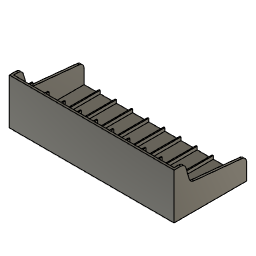
Oblig2Fusion360 (Autodesk Fusion 360 design; units mm, degrees)
Autodesk Fusion 360 part; units mm, degrees
note: some values were not read from the file. Chosen so that the rebuilt part matches the saved one: which face or edge a step refers to. Set by a fixed rule: which sketch regions a step uses.
sketch "Sketch1" plane through (0, 0, 0) normal (0, 0, 1) x (1, 0, 0)
  line L0 (2, 2) -> (172, 2)
  line L1 (172, 2) -> (172, 137)
  line L2 (172, 137) -> (2, 137)
  line L3 (2, 137) -> (2, 2)
  dimension "d1" = 170
  dimension "d2" = 135
  constraint horizontal L0
  constraint vertical L1
  constraint horizontal L2
  constraint vertical L3
  measures "d1" distance of L0.start L0.end
  measures "d2" distance of L0.start L2.end
sketch "Sketch2" plane through (0, 0, 0) normal (0, 0, 1) x (1, 0, 0)
  line L0 (10, 10) -> (158, 10)
  line L1 (158, 10) -> (158, 77.5)
  line L2 (158, 77.5) -> (10, 77.5)
  line L3 (10, 77.5) -> (10, 10)
  dimension "d5" = 148
  dimension "d6" = 67.5
  constraint horizontal L0
  constraint vertical L1
  constraint horizontal L2
  constraint vertical L3
  measures "d5" distance of L0.start L0.end
  measures "d6" distance of L0.start L2.end
extrude "Extrude2" add sketch "Sketch2" along normal blind 42.5
sketch "Sketch3" plane through (158, 0, 0) normal (1, 0, 0) x (0, 1, 0)
  line L0 (10, 0) -> (77.5, 0)
  line L1 (77.5, 0) -> (77.5, 42.5)
  line L2 (77.5, 42.5) -> (10, 42.5)
  line L3 (10, 42.5) -> (10, 0)
  line L4 (10, 42.5) -> (16.2285, 42.5)
  line L5 (28.3819, 24.6655) -> (72.9921, 20.2531)
  line L6 (24.0664, 28.2676) -> (21.0361, 38.8736)
  line L7 (10, 42.5) -> (10, 0)
  line L8 (77.5, 0) -> (77.5, 15.2774)
  line L9 (77.5, 0) -> (10, 0)
  arc A0 (77.5, 15.2774) -> (72.9921, 20.2531) centre (72.5, 15.2774) ccw
  arc A1 (21.0361, 38.8736) -> (16.2285, 42.5) centre (16.2285, 37.5) ccw
  arc A2 (24.0664, 28.2676) -> (28.3819, 24.6655) centre (28.874, 29.6412) ccw
  dimension "d9" = 5
  constraint coincident L2.end L3.start
  constraint perpendicular L3 L4
  constraint coincident L0.start L3.end
  constraint coincident L0.end L1.start
  constraint tangent L5 A0
  constraint tangent L8 A0
  constraint tangent L4 A1
  constraint tangent L6 A1
  constraint equal A0 A1
  constraint tangent L6 A2
  constraint tangent L5 A2
  constraint equal A0 A2
  measures "d9" radius of A0
extrude "Extrude3" cut sketch "Sketch3" against normal blind 150 contours L1 L2 L5 L6 A0 A1 A2
extrude "Extrude4" add 1 faces at (158, 38.6273, 8.2218) along direction (1, 0, 0) blind 4
sketch "Sketch4" plane through (0, 77.5, 0) normal (0, 1, 0) x (-1, 0, 0)
  line L0 (-10, 15.2774) -> (-162, 15.2774)
  line L1 (-162, 15.2774) -> (-162, 0)
  line L2 (-162, 0) -> (-10, 0)
  line L3 (-10, 0) -> (-10, 15.2774)
  line L4 (-162, 15.2774) -> (-160, 15.2774)
  line L5 (-160, 15.2774) -> (-160, 0)
  line L6 (-160, 0) -> (-162, 0)
  line L7 (-162, 0) -> (-162, 15.2774)
  line L8 (-162, 15.2774) -> (-160, 15.2774)
  line L9 (-160, 15.2774) -> (-160, 86.9563)
  line L10 (-160, 86.9563) -> (-162, 86.9563)
  line L11 (-162, 86.9563) -> (-162, 15.2774)
  line L12 (-10, 0) -> (-12, 0)
  line L13 (-12, 0) -> (-12, 80)
  line L14 (-12, 80) -> (-10, 80)
  line L15 (-10, 80) -> (-10, 0)
  line L16 (-160, 0) -> (-12, 0)
  line L17 (-12, 0) -> (-12, 80)
  line L18 (-12, 80) -> (-160, 80)
  line L19 (-160, 80) -> (-160, 0)
  dimension "d14" = 2
  constraint horizontal L4
  constraint vertical L5
  constraint horizontal L6
  constraint vertical L7
  constraint coincident L0.end L1.start
  constraint horizontal L8
  constraint vertical L9
  constraint horizontal L10
  constraint vertical L11
  constraint horizontal L12
  constraint vertical L13
  constraint horizontal L14
  constraint vertical L15
  constraint coincident L2.end L3.start
  constraint horizontal L16
  constraint vertical L17
  constraint horizontal L18
  constraint vertical L19
  measures "d14" distance of L0.end L4.end
extrude "Extrude5" cut sketch "Sketch4" against normal blind 65.5 contours L0 L9 L13 L17 L18 L19
sketch "Sketch5" plane through (0, 77.5, 0) normal (0, 1, 0) x (-1, 0, 0)
  line L0 (-10, 15.2774) -> (-12, 15.2774)
  line L1 (-12, 15.2774) -> (-160, 15.2774)
  line L2 (-160, 15.2774) -> (-162, 15.2774)
  line L3 (-162, 15.2774) -> (-162, 0)
  line L4 (-162, 0) -> (-10, 0)
  line L5 (-10, 0) -> (-10, 15.2774)
  line L6 (-162, 15.2774) -> (-160, 15.2774)
  line L7 (-160, 15.2774) -> (-160, 0)
  line L8 (-160, 0) -> (-162, 0)
  line L9 (-162, 0) -> (-162, 15.2774)
  line L10 (-10, 15.2774) -> (-12, 15.2774)
  line L11 (-12, 15.2774) -> (-12, 0)
  line L12 (-12, 0) -> (-10, 0)
  line L13 (-10, 0) -> (-10, 15.2774)
  line L14 (-160, 15.2774) -> (-12, 15.2774)
  line L15 (-12, 15.2774) -> (-12, 0)
  line L16 (-12, 0) -> (-160, 0)
  line L17 (-160, 0) -> (-160, 15.2774)
  constraint horizontal L6
  constraint vertical L7
  constraint horizontal L8
  constraint vertical L9
  constraint coincident L4 L7.end
  constraint coincident L2.end L3.start
  constraint horizontal L10
  constraint vertical L11
  constraint horizontal L12
  constraint vertical L13
  constraint coincident L4 L11.end
  constraint coincident L0.start L5.end
  constraint horizontal L14
  constraint vertical L15
  constraint horizontal L16
  constraint vertical L17
  constraint coincident L1.end L2.start
extrude "Extrude6" cut sketch "Sketch5" against normal blind 65.5 contours L1 L4 L7 L11 L14 L15 L16 L17
sketch "Sketch6" plane through (0, 0, 0) normal (0, 0, 1) x (1, 0, 0)
  line L0 (12, 12) -> (160, 12)
  line L1 (160, 12) -> (160, 77.5)
  line L2 (160, 77.5) -> (12, 77.5)
  line L3 (12, 77.5) -> (12, 12)
  constraint horizontal L0
  constraint vertical L1
  constraint horizontal L2
  constraint vertical L3
extrude "Extrude7" add sketch "Sketch6" along normal blind 2
extrude "Extrude8" add 1 faces at (61.3333, 55.6667, 2) along direction (0, 0, 1) blind 3
sketch "Sketch7" plane through (0, 0, 5) normal (0, 0, 1) x (-1, 0, 0)
  line L0 (-12, -77.5) -> (-12, -12)
  line L1 (-12, -12) -> (-160, -12)
  line L2 (-160, -12) -> (-160, -77.5)
  line L3 (-160, -77.5) -> (-12, -77.5)
  line L4 (-160, -77.5) -> (-146, -77.5)
  line L5 (-146, -77.5) -> (-146, -12)
  line L6 (-146, -12) -> (-160, -12)
  line L7 (-160, -12) -> (-160, -77.5)
  dimension "d24" = 14
  dimension "d25" = 65.5
  constraint horizontal L4
  constraint vertical L5
  constraint horizontal L6
  constraint vertical L7
  constraint coincident L2.end L3.start
  measures "d24" distance of L2.end L4.end
  measures "d25" distance of L2.end L1.end
extrude "Extrude9" cut sketch "Sketch7" against normal blind 3 contours L1 L2 L3 L4 L5 L6 L7
sketch "Sketch8" plane through (0, 0, 5) normal (0, 0, 1) x (-1, 0, 0)
  line L0 (-146, -12) -> (-146, -77.5)
  line L1 (-146, -77.5) -> (-12, -77.5)
  line L2 (-12, -77.5) -> (-12, -12)
  line L3 (-12, -12) -> (-146, -12)
  line L4 (-146, -77.5) -> (-145, -77.5)
  line L5 (-145, -77.5) -> (-145, -12)
  line L6 (-145, -12) -> (-146, -12)
  line L7 (-146, -12) -> (-146, -77.5)
  line L8 (-145, -77.5) -> (-131, -77.5)
  line L9 (-131, -77.5) -> (-131, -12)
  line L10 (-131, -12) -> (-145, -12)
  line L11 (-145, -12) -> (-145, -77.5)
  line L12 (-131, -77.5) -> (-130, -77.5)
  line L13 (-130, -77.5) -> (-130, -12)
  line L14 (-130, -12) -> (-131, -12)
  line L15 (-131, -12) -> (-131, -77.5)
  dimension "d28" = 1
  dimension "d29" = 65.5
  dimension "d30" = 14
  dimension "d31" = 65.5
  dimension "d32" = 1
  dimension "d33" = 65.5
  constraint horizontal L4
  constraint vertical L5
  constraint horizontal L6
  constraint vertical L7
  constraint coincident L0.end L1.start
  constraint horizontal L8
  constraint vertical L9
  constraint horizontal L10
  constraint vertical L11
  constraint horizontal L12
  constraint vertical L13
  constraint horizontal L14
  constraint vertical L15
  measures "d28" distance of L0.end L4.end
  measures "d29" distance of L0.end L0.start
  measures "d30" distance of L4.end L8.end
  measures "d31" distance of L4.end L5.end
  measures "d32" distance of L8.end L12.end
  measures "d33" distance of L8.end L9.end
extrude "Extrude10" cut sketch "Sketch8" against normal blind 3 contours L1 L3 L5 L8 L9 L10 L11 L15
sketch "Sketch9" plane through (0, 0, 5) normal (0, 0, 1) x (-1, 0, 0)
  line L0 (-131, -12) -> (-131, -77.5)
  line L1 (-131, -77.5) -> (-12, -77.5)
  line L2 (-12, -77.5) -> (-12, -12)
  line L3 (-12, -12) -> (-131, -12)
  line L4 (-12, -77.5) -> (-26, -77.5)
  line L5 (-26, -77.5) -> (-26, -12)
  line L6 (-26, -12) -> (-12, -12)
  line L7 (-12, -12) -> (-12, -77.5)
  line L8 (-26, -77.5) -> (-27, -77.5)
  line L9 (-27, -77.5) -> (-27, -12)
  line L10 (-27, -12) -> (-26, -12)
  line L11 (-26, -12) -> (-26, -77.5)
  line L12 (-27, -77.5) -> (-41, -77.5)
  line L13 (-41, -77.5) -> (-41, -12)
  line L14 (-41, -12) -> (-27, -12)
  line L15 (-27, -12) -> (-27, -77.5)
  line L16 (-41, -77.5) -> (-42, -77.5)
  line L17 (-42, -77.5) -> (-42, -12)
  line L18 (-42, -12) -> (-41, -12)
  line L19 (-41, -12) -> (-41, -77.5)
  line L20 (-42, -77.5) -> (-56, -77.5)
  line L21 (-56, -77.5) -> (-56, -12)
  line L22 (-56, -12) -> (-42, -12)
  line L23 (-42, -12) -> (-42, -77.5)
  line L24 (-56, -77.5) -> (-57, -77.5)
  line L25 (-57, -77.5) -> (-57, -12)
  line L26 (-57, -12) -> (-56, -12)
  line L27 (-56, -12) -> (-56, -77.5)
  line L28 (-57, -77.5) -> (-71, -77.5)
  line L29 (-71, -77.5) -> (-71, -12)
  line L30 (-71, -12) -> (-57, -12)
  line L31 (-57, -12) -> (-57, -77.5)
  line L32 (-71, -77.5) -> (-72, -77.5)
  line L33 (-72, -77.5) -> (-72, -12)
  line L34 (-72, -12) -> (-71, -12)
  line L35 (-71, -12) -> (-71, -77.5)
  line L36 (-72, -77.5) -> (-86, -77.5)
  line L37 (-86, -77.5) -> (-86, -12)
  line L38 (-86, -12) -> (-72, -12)
  line L39 (-72, -12) -> (-72, -77.5)
  line L40 (-86, -77.5) -> (-87, -77.5)
  line L41 (-87, -77.5) -> (-87, -12)
  line L42 (-87, -12) -> (-86, -12)
  line L43 (-86, -12) -> (-86, -77.5)
  line L44 (-87, -77.5) -> (-101, -77.5)
  line L45 (-101, -77.5) -> (-101, -12)
  line L46 (-101, -12) -> (-87, -12)
  line L47 (-87, -12) -> (-87, -77.5)
  line L48 (-101, -77.5) -> (-102, -77.5)
  line L49 (-102, -77.5) -> (-102, -12)
  line L50 (-102, -12) -> (-101, -12)
  line L51 (-101, -12) -> (-101, -77.5)
  line L52 (-102, -77.5) -> (-116, -77.5)
  line L53 (-116, -77.5) -> (-116, -12)
  line L54 (-116, -12) -> (-102, -12)
  line L55 (-102, -12) -> (-102, -77.5)
  line L56 (-116, -77.5) -> (-117, -77.5)
  line L57 (-117, -77.5) -> (-117, -12)
  line L58 (-117, -12) -> (-116, -12)
  line L59 (-116, -12) -> (-116, -77.5)
  line L60 (-117, -77.5) -> (-131, -77.5)
  line L61 (-131, -77.5) -> (-131, -12)
  line L62 (-131, -12) -> (-117, -12)
  line L63 (-117, -12) -> (-117, -77.5)
  dimension "d36" = 14
  dimension "d37" = 65.5
  dimension "d38" = 1
  dimension "d39" = 65.5
  dimension "d40" = 14
  dimension "d41" = 65.5
  dimension "d42" = 1
  dimension "d43" = 65.5
  dimension "d44" = 14
  dimension "d45" = 65.5
  dimension "d46" = 1
  dimension "d47" = 65.5
  dimension "d48" = 14
  dimension "d49" = 65.5
  dimension "d50" = 1
  dimension "d51" = 65.5
  dimension "d52" = 14
  dimension "d53" = 65.5
  dimension "d54" = 1
  dimension "d55" = 65.5
  dimension "d56" = 14
  dimension "d57" = 65.5
  dimension "d58" = 1
  dimension "d59" = 65.5
  dimension "d60" = 14
  dimension "d61" = 65.5
  dimension "d62" = 1
  dimension "d63" = 65.5
  dimension "d64" = 14
  dimension "d65" = 65.5
  constraint horizontal L4
  constraint vertical L5
  constraint horizontal L6
  constraint vertical L7
  constraint coincident L1.end L2.start
  constraint horizontal L8
  constraint vertical L9
  constraint horizontal L10
  constraint vertical L11
  constraint horizontal L12
  constraint vertical L13
  constraint horizontal L14
  constraint vertical L15
  constraint horizontal L16
  constraint vertical L17
  constraint horizontal L18
  constraint vertical L19
  constraint horizontal L20
  constraint vertical L21
  constraint horizontal L22
  constraint vertical L23
  constraint horizontal L24
  constraint vertical L25
  constraint horizontal L26
  constraint vertical L27
  constraint horizontal L28
  constraint vertical L29
  constraint horizontal L30
  constraint vertical L31
  constraint horizontal L32
  constraint vertical L33
  constraint horizontal L34
  constraint vertical L35
  constraint horizontal L36
  constraint vertical L37
  constraint horizontal L38
  constraint vertical L39
  constraint horizontal L40
  constraint vertical L41
  constraint horizontal L42
  constraint vertical L43
  constraint horizontal L44
  constraint vertical L45
  constraint horizontal L46
  constraint vertical L47
  constraint horizontal L48
  constraint vertical L49
  constraint horizontal L50
  constraint vertical L51
  constraint horizontal L52
  constraint vertical L53
  constraint horizontal L54
  constraint vertical L55
  constraint horizontal L56
  constraint vertical L57
  constraint horizontal L58
  constraint vertical L59
  constraint horizontal L60
  constraint vertical L61
  constraint horizontal L62
  constraint vertical L63
  measures "d36" distance of L1.end L4.end
  measures "d37" distance of L1.end L2.end
  measures "d38" distance of L4.end L8.end
  measures "d39" distance of L4.end L5.end
  measures "d40" distance of L8.end L12.end
  measures "d41" distance of L8.end L9.end
  measures "d42" distance of L12.end L16.end
  measures "d43" distance of L12.end L13.end
  measures "d44" distance of L16.end L20.end
  measures "d45" distance of L16.end L17.end
  measures "d46" distance of L20.end L24.end
  measures "d47" distance of L20.end L21.end
  measures "d48" distance of L24.end L28.end
  measures "d49" distance of L24.end L25.end
  measures "d50" distance of L28.end L32.end
  measures "d51" distance of L28.end L29.end
  measures "d52" distance of L32.end L36.end
  measures "d53" distance of L32.end L33.end
  measures "d54" distance of L36.end L40.end
  measures "d55" distance of L36.end L37.end
  measures "d56" distance of L40.end L44.end
  measures "d57" distance of L40.end L41.end
  measures "d58" distance of L44.end L48.end
  measures "d59" distance of L44.end L45.end
  measures "d60" distance of L48.end L52.end
  measures "d61" distance of L48.end L49.end
  measures "d62" distance of L52.end L56.end
  measures "d63" distance of L52.end L53.end
  measures "d64" distance of L56.end L0.end
  measures "d65" distance of L56.end L57.end
extrude "Extrude11" add 1 faces at (162, 38.6273, 8.2218) along direction (1, 0, 0) blind 1
sketch "Sketch10" plane through (160, 0, 0) normal (-1, 0, 0) x (0, -1, 0)
  line L0 (-12, 5) -> (-12, 42.5)
  line L1 (-12, 42.5) -> (-16.2285, 42.5)
  arc A0 (-16.2285, 42.5) -> (-21.0361, 38.8736) centre (-16.2285, 37.5) ccw
  line L2 (-21.0361, 38.8736) -> (-24.0664, 28.2676)
  arc A1 (-28.3819, 24.6655) -> (-24.0664, 28.2676) centre (-28.874, 29.6412) ccw
  line L3 (-28.3819, 24.6655) -> (-72.9921, 20.2531)
  arc A2 (-72.9921, 20.2531) -> (-77.5, 15.2774) centre (-72.5, 15.2774) ccw
  line L4 (-77.5, 15.2774) -> (-77.5, 5)
  line L5 (-77.5, 5) -> (-77.5, 2)
  line L6 (-77.5, 2) -> (-12, 2)
  line L7 (-12, 2) -> (-12, 5)
extrude "Extrude12" cut sketch "Sketch10" against normal blind 1
extrude "Extrude13" add 1 faces at (146, 55.6667, 4) along direction (1, 0, 0) blind 1
extrude "Extrude14" cut 1 faces at (145, 55.6667, 4) along direction (1, 0, 0) blind 1
extrude "Extrude15" add 1 faces at (131, 55.6667, 4) along direction (1, 0, 0) blind 1
extrude "Extrude16" cut sketch "Sketch9" against normal blind 3 contours L0 L1 L3 L57 L60 L61 L62 L63
sketch "Sketch11" plane through (0, 0, 5) normal (0, 0, 1) x (-1, 0, 0)
  line L0 (-117, -12) -> (-117, -77.5)
  line L1 (-117, -77.5) -> (-12, -77.5)
  line L2 (-12, -77.5) -> (-12, -12)
  line L3 (-12, -12) -> (-117, -12)
  line L4 (-117, -77.5) -> (-116, -77.5)
  line L5 (-116, -77.5) -> (-116, -12)
  line L6 (-116, -12) -> (-117, -12)
  line L7 (-117, -12) -> (-117, -77.5)
  line L8 (-116, -77.5) -> (-102, -77.5)
  line L9 (-102, -77.5) -> (-102, -12)
  line L10 (-102, -12) -> (-116, -12)
  line L11 (-116, -12) -> (-116, -77.5)
  dimension "d78" = 1
  dimension "d79" = 65.5
  dimension "d80" = 14
  dimension "d81" = 65.5
  constraint horizontal L4
  constraint vertical L5
  constraint horizontal L6
  constraint vertical L7
  constraint coincident L0.end L1.start
  constraint horizontal L8
  constraint vertical L9
  constraint horizontal L10
  constraint vertical L11
  measures "d78" distance of L0.end L4.end
  measures "d79" distance of L0.end L0.start
  measures "d80" distance of L4.end L8.end
  measures "d81" distance of L4.end L5.end
extrude "Extrude17" cut sketch "Sketch11" against normal blind 3 contours L1 L3 L5 L8 L9 L10 L11
sketch "Sketch12" plane through (0, 0, 5) normal (0, 0, 1) x (-1, 0, 0)
  line L0 (-102, -12) -> (-102, -77.5)
  line L1 (-102, -77.5) -> (-12, -77.5)
  line L2 (-12, -77.5) -> (-12, -12)
  line L3 (-12, -12) -> (-102, -12)
  line L4 (-102, -77.5) -> (-101, -77.5)
  line L5 (-101, -77.5) -> (-101, -12)
  line L6 (-101, -12) -> (-102, -12)
  line L7 (-102, -12) -> (-102, -77.5)
  line L8 (-101, -77.5) -> (-87, -77.5)
  line L9 (-87, -77.5) -> (-87, -12)
  line L10 (-87, -12) -> (-101, -12)
  line L11 (-101, -12) -> (-101, -77.5)
  dimension "d84" = 1
  dimension "d85" = 65.5
  dimension "d86" = 14
  dimension "d87" = 65.5
  constraint horizontal L4
  constraint vertical L5
  constraint horizontal L6
  constraint vertical L7
  constraint coincident L0.end L1.start
  constraint horizontal L8
  constraint vertical L9
  constraint horizontal L10
  constraint vertical L11
  measures "d84" distance of L0.end L4.end
  measures "d85" distance of L0.end L0.start
  measures "d86" distance of L4.end L8.end
  measures "d87" distance of L4.end L5.end
extrude "Extrude18" cut sketch "Sketch12" against normal blind 3 contours L1 L3 L5 L8 L9 L10 L11
sketch "Sketch13" plane through (0, 0, 5) normal (0, 0, 1) x (-1, 0, 0)
  line L0 (-87, -12) -> (-87, -77.5)
  line L1 (-87, -77.5) -> (-12, -77.5)
  line L2 (-12, -77.5) -> (-12, -12)
  line L3 (-12, -12) -> (-87, -12)
  line L4 (-87, -77.5) -> (-86, -77.5)
  line L5 (-86, -77.5) -> (-86, -12)
  line L6 (-86, -12) -> (-87, -12)
  line L7 (-87, -12) -> (-87, -77.5)
  line L8 (-86, -77.5) -> (-72, -77.5)
  line L9 (-72, -77.5) -> (-72, -12)
  line L10 (-72, -12) -> (-86, -12)
  line L11 (-86, -12) -> (-86, -77.5)
  dimension "d90" = 1
  dimension "d91" = 65.5
  dimension "d92" = 14
  dimension "d93" = 65.5
  constraint horizontal L4
  constraint vertical L5
  constraint horizontal L6
  constraint vertical L7
  constraint coincident L0.end L1.start
  constraint horizontal L8
  constraint vertical L9
  constraint horizontal L10
  constraint vertical L11
  measures "d90" distance of L0.end L4.end
  measures "d91" distance of L0.end L0.start
  measures "d92" distance of L4.end L8.end
  measures "d93" distance of L4.end L5.end
extrude "Extrude19" cut sketch "Sketch13" against normal blind 3 contours L1 L3 L5 L8 L9 L10 L11
sketch "Sketch14" plane through (0, 0, 5) normal (0, 0, 1) x (-1, 0, 0)
  line L0 (-72, -12) -> (-72, -77.5)
  line L1 (-72, -77.5) -> (-12, -77.5)
  line L2 (-12, -77.5) -> (-12, -12)
  line L3 (-12, -12) -> (-72, -12)
  line L4 (-72, -77.5) -> (-71, -77.5)
  line L5 (-71, -77.5) -> (-71, -12)
  line L6 (-71, -12) -> (-72, -12)
  line L7 (-72, -12) -> (-72, -77.5)
  line L8 (-71, -77.5) -> (-57, -77.5)
  line L9 (-57, -77.5) -> (-57, -12)
  line L10 (-57, -12) -> (-71, -12)
  line L11 (-71, -12) -> (-71, -77.5)
  dimension "d96" = 1
  dimension "d97" = 65.5
  dimension "d98" = 14
  dimension "d99" = 65.5
  constraint horizontal L4
  constraint vertical L5
  constraint horizontal L6
  constraint vertical L7
  constraint coincident L0.end L1.start
  constraint horizontal L8
  constraint vertical L9
  constraint horizontal L10
  constraint vertical L11
  measures "d96" distance of L0.end L4.end
  measures "d97" distance of L0.end L0.start
  measures "d98" distance of L4.end L8.end
  measures "d99" distance of L4.end L5.end
extrude "Extrude20" cut sketch "Sketch14" against normal blind 3 contours L1 L3 L5 L8 L9 L10 L11
sketch "Sketch15" plane through (0, 0, 5) normal (0, 0, 1) x (-1, 0, 0)
  line L0 (-57, -12) -> (-57, -77.5)
  line L1 (-57, -77.5) -> (-12, -77.5)
  line L2 (-12, -77.5) -> (-12, -12)
  line L3 (-12, -12) -> (-57, -12)
  line L4 (-57, -77.5) -> (-56, -77.5)
  line L5 (-56, -77.5) -> (-56, -12)
  line L6 (-56, -12) -> (-57, -12)
  line L7 (-57, -12) -> (-57, -77.5)
  line L8 (-56, -77.5) -> (-42, -77.5)
  line L9 (-42, -77.5) -> (-42, -12)
  line L10 (-42, -12) -> (-56, -12)
  line L11 (-56, -12) -> (-56, -77.5)
  dimension "d102" = 1
  dimension "d103" = 65.5
  dimension "d104" = 14
  dimension "d105" = 65.5
  constraint horizontal L4
  constraint vertical L5
  constraint horizontal L6
  constraint vertical L7
  constraint coincident L0.end L1.start
  constraint horizontal L8
  constraint vertical L9
  constraint horizontal L10
  constraint vertical L11
  measures "d102" distance of L0.end L4.end
  measures "d103" distance of L0.end L0.start
  measures "d104" distance of L4.end L8.end
  measures "d105" distance of L4.end L5.end
extrude "Extrude21" cut sketch "Sketch15" against normal blind 3 contours L1 L3 L5 L8 L9 L10 L11
sketch "Sketch16" plane through (0, 0, 5) normal (0, 0, 1) x (-1, 0, 0)
  line L0 (-42, -12) -> (-42, -77.5)
  line L1 (-42, -77.5) -> (-12, -77.5)
  line L2 (-12, -77.5) -> (-12, -12)
  line L3 (-12, -12) -> (-42, -12)
  line L4 (-42, -77.5) -> (-41, -77.5)
  line L5 (-41, -77.5) -> (-41, -12)
  line L6 (-41, -12) -> (-42, -12)
  line L7 (-42, -12) -> (-42, -77.5)
  line L8 (-41, -77.5) -> (-27, -77.5)
  line L9 (-27, -77.5) -> (-27, -12)
  line L10 (-27, -12) -> (-41, -12)
  line L11 (-41, -12) -> (-41, -77.5)
  dimension "d108" = 1
  dimension "d109" = 65.5
  dimension "d110" = 14
  dimension "d111" = 65.5
  constraint horizontal L4
  constraint vertical L5
  constraint horizontal L6
  constraint vertical L7
  constraint coincident L0.end L1.start
  constraint horizontal L8
  constraint vertical L9
  constraint horizontal L10
  constraint vertical L11
  measures "d108" distance of L0.end L4.end
  measures "d109" distance of L0.end L0.start
  measures "d110" distance of L4.end L8.end
  measures "d111" distance of L4.end L5.end
extrude "Extrude22" cut sketch "Sketch16" against normal blind 3 contours L1 L3 L5 L8 L9 L10 L11
sketch "Sketch17" plane through (0, 0, 5) normal (0, 0, 1) x (-1, 0, 0)
  line L0 (-27, -12) -> (-27, -77.5)
  line L1 (-27, -77.5) -> (-12, -77.5)
  line L2 (-12, -77.5) -> (-12, -12)
  line L3 (-12, -12) -> (-27, -12)
  line L4 (-12, -77.5) -> (-26, -77.5)
  line L5 (-26, -77.5) -> (-26, -12)
  line L6 (-26, -12) -> (-12, -12)
  line L7 (-12, -12) -> (-12, -77.5)
  dimension "d114" = 14
  dimension "d115" = 65.5
  constraint horizontal L4
  constraint vertical L5
  constraint horizontal L6
  constraint vertical L7
  constraint coincident L1.end L2.start
  measures "d114" distance of L1.end L4.end
  measures "d115" distance of L1.end L2.end
extrude "Extrude23" cut sketch "Sketch17" against normal blind 3 contours L1 L2 L3 L4 L5 L6 L7
sketch "Sketch18" plane through (0, 12, 0) normal (0, 1, 0) x (-1, 0, 0)
  line L0 (-132, 5) -> (-131, 5)
  line L1 (-131, 5) -> (-131, 2)
  line L2 (-131, 2) -> (-117, 2)
  line L3 (-117, 2) -> (-117, 5)
  line L4 (-117, 5) -> (-116, 5)
  line L5 (-116, 5) -> (-116, 2)
  line L6 (-116, 2) -> (-102, 2)
  line L7 (-102, 2) -> (-102, 5)
  line L8 (-102, 5) -> (-101, 5)
  line L9 (-101, 5) -> (-101, 2)
  line L10 (-101, 2) -> (-87, 2)
  line L11 (-87, 2) -> (-87, 5)
  line L12 (-87, 5) -> (-86, 5)
  line L13 (-86, 5) -> (-86, 2)
  line L14 (-86, 2) -> (-72, 2)
  line L15 (-72, 2) -> (-72, 5)
  line L16 (-72, 5) -> (-71, 5)
  line L17 (-71, 5) -> (-71, 2)
  line L18 (-71, 2) -> (-57, 2)
  line L19 (-57, 2) -> (-57, 5)
  line L20 (-57, 5) -> (-56, 5)
  line L21 (-56, 5) -> (-56, 2)
  line L22 (-56, 2) -> (-42, 2)
  line L23 (-42, 2) -> (-42, 5)
  line L24 (-42, 5) -> (-41, 5)
  line L25 (-41, 5) -> (-41, 2)
  line L26 (-41, 2) -> (-27, 2)
  line L27 (-27, 2) -> (-27, 5)
  line L28 (-27, 5) -> (-26, 5)
  line L29 (-26, 5) -> (-26, 2)
  line L30 (-26, 2) -> (-12, 2)
  line L31 (-12, 2) -> (-12, 42.5)
  line L32 (-12, 42.5) -> (-161, 42.5)
  line L33 (-161, 42.5) -> (-161, 2)
  line L34 (-161, 2) -> (-147, 2)
  line L35 (-147, 2) -> (-147, 5)
  line L36 (-147, 5) -> (-146, 5)
  line L37 (-146, 5) -> (-146, 2)
  line L38 (-146, 2) -> (-132, 2)
  line L39 (-132, 2) -> (-132, 5)
  line L40 (-161, 42.5) -> (-12, 42.5)
  line L41 (-12, 42.5) -> (-12, 2)
  line L42 (-12, 2) -> (-161, 2)
  line L43 (-161, 2) -> (-161, 42.5)
  constraint horizontal L40
  constraint vertical L41
  constraint horizontal L42
  constraint vertical L43
  constraint coincident L30.end L31.start
  constraint coincident L32.end L33.start
extrude "Extrude24" add sketch "Sketch18" along normal blind 3 contours L0 L1 L2 L3 L4 L5 L6 L7 L8 L9 L10 L11 L12 L13 L14 L15 L16 L17 L18 L19 L20 L21 L22 L23 L24 L25 L26 L27 L28 L29 L30 L31 L32 L33 L34 L35 L36 L37 L38 L39 L40 L41 L42 L43
extrude "Extrude25" add 1 faces at (161, 40.294, 9.5552) along direction (1, 0, 0) blind 1
extrude "Extrude26" cut 1 faces at (86.3333, 15, 30) along direction (0, -1, 0) blind 3
sketch "Sketch19" plane through (0, 12, 0) normal (0, 1, 0) x (-1, 0, 0)
  line L0 (-161, 42.5) -> (-161, 2)
  line L1 (-161, 2) -> (-147, 2)
  line L2 (-147, 2) -> (-147, 5)
  line L3 (-147, 5) -> (-146, 5)
  line L4 (-146, 5) -> (-146, 2)
  line L5 (-146, 2) -> (-132, 2)
  line L6 (-132, 2) -> (-132, 5)
  line L7 (-132, 5) -> (-131, 5)
  line L8 (-131, 5) -> (-131, 2)
  line L9 (-131, 2) -> (-117, 2)
  line L10 (-117, 2) -> (-117, 5)
  line L11 (-117, 5) -> (-116, 5)
  line L12 (-116, 5) -> (-116, 2)
  line L13 (-116, 2) -> (-102, 2)
  line L14 (-102, 2) -> (-102, 5)
  line L15 (-102, 5) -> (-101, 5)
  line L16 (-101, 5) -> (-101, 2)
  line L17 (-101, 2) -> (-87, 2)
  line L18 (-87, 2) -> (-87, 5)
  line L19 (-87, 5) -> (-86, 5)
  line L20 (-86, 5) -> (-86, 2)
  line L21 (-86, 2) -> (-72, 2)
  line L22 (-72, 2) -> (-72, 5)
  line L23 (-72, 5) -> (-71, 5)
  line L24 (-71, 5) -> (-71, 2)
  line L25 (-71, 2) -> (-57, 2)
  line L26 (-57, 2) -> (-57, 5)
  line L27 (-57, 5) -> (-56, 5)
  line L28 (-56, 5) -> (-56, 2)
  line L29 (-56, 2) -> (-42, 2)
  line L30 (-42, 2) -> (-42, 5)
  line L31 (-42, 5) -> (-41, 5)
  line L32 (-41, 5) -> (-41, 2)
  line L33 (-41, 2) -> (-27, 2)
  line L34 (-27, 2) -> (-27, 5)
  line L35 (-27, 5) -> (-26, 5)
  line L36 (-26, 5) -> (-26, 2)
  line L37 (-26, 2) -> (-12, 2)
  line L38 (-12, 2) -> (-12, 42.5)
  line L39 (-12, 42.5) -> (-161, 42.5)
  line L40 (-147, 5) -> (-146, 5)
  line L41 (-146, 5) -> (-146, 42.5)
  line L42 (-146, 42.5) -> (-147, 42.5)
  line L43 (-147, 42.5) -> (-147, 5)
  dimension "d124" = 1
  constraint horizontal L40
  constraint vertical L41
  constraint horizontal L42
  constraint vertical L43
  constraint coincident L39 L41.end
  constraint coincident L2.end L3.start
  measures "d124" distance of L2.end L3.end
extrude "Extrude27" add sketch "Sketch19" along normal blind 3 contours L3 L39 L40 L41 L42 L43
sketch "Sketch20" plane through (0, 12, 0) normal (0, 1, 0) x (-1, 0, 0)
  line L0 (-146, 42.5) -> (-146, 2)
  line L1 (-146, 2) -> (-132, 2)
  line L2 (-132, 2) -> (-132, 5)
  line L3 (-132, 5) -> (-131, 5)
  line L4 (-131, 5) -> (-131, 2)
  line L5 (-131, 2) -> (-117, 2)
  line L6 (-117, 2) -> (-117, 5)
  line L7 (-117, 5) -> (-116, 5)
  line L8 (-116, 5) -> (-116, 2)
  line L9 (-116, 2) -> (-102, 2)
  line L10 (-102, 2) -> (-102, 5)
  line L11 (-102, 5) -> (-101, 5)
  line L12 (-101, 5) -> (-101, 2)
  line L13 (-101, 2) -> (-87, 2)
  line L14 (-87, 2) -> (-87, 5)
  line L15 (-87, 5) -> (-86, 5)
  line L16 (-86, 5) -> (-86, 2)
  line L17 (-86, 2) -> (-72, 2)
  line L18 (-72, 2) -> (-72, 5)
  line L19 (-72, 5) -> (-71, 5)
  line L20 (-71, 5) -> (-71, 2)
  line L21 (-71, 2) -> (-57, 2)
  line L22 (-57, 2) -> (-57, 5)
  line L23 (-57, 5) -> (-56, 5)
  line L24 (-56, 5) -> (-56, 2)
  line L25 (-56, 2) -> (-42, 2)
  line L26 (-42, 2) -> (-42, 5)
  line L27 (-42, 5) -> (-41, 5)
  line L28 (-41, 5) -> (-41, 2)
  line L29 (-41, 2) -> (-27, 2)
  line L30 (-27, 2) -> (-27, 5)
  line L31 (-27, 5) -> (-26, 5)
  line L32 (-26, 5) -> (-26, 2)
  line L33 (-26, 2) -> (-12, 2)
  line L34 (-12, 2) -> (-12, 42.5)
  line L35 (-12, 42.5) -> (-146, 42.5)
  line L36 (-132, 5) -> (-131, 5)
  line L37 (-131, 5) -> (-131, 42.5)
  line L38 (-131, 42.5) -> (-132, 42.5)
  line L39 (-132, 42.5) -> (-132, 5)
  constraint horizontal L36
  constraint vertical L37
  constraint horizontal L38
  constraint vertical L39
  constraint coincident L35 L37.end
  constraint coincident L2.end L3.start
extrude "Extrude28" add sketch "Sketch20" along normal blind 3 contours L3 L35 L36 L37 L38 L39
sketch "Sketch21" plane through (0, 12, 0) normal (0, 1, 0) x (-1, 0, 0)
  line L0 (-131, 42.5) -> (-131, 2)
  line L1 (-131, 2) -> (-117, 2)
  line L2 (-117, 2) -> (-117, 5)
  line L3 (-117, 5) -> (-116, 5)
  line L4 (-116, 5) -> (-116, 2)
  line L5 (-116, 2) -> (-102, 2)
  line L6 (-102, 2) -> (-102, 5)
  line L7 (-102, 5) -> (-101, 5)
  line L8 (-101, 5) -> (-101, 2)
  line L9 (-101, 2) -> (-87, 2)
  line L10 (-87, 2) -> (-87, 5)
  line L11 (-87, 5) -> (-86, 5)
  line L12 (-86, 5) -> (-86, 2)
  line L13 (-86, 2) -> (-72, 2)
  line L14 (-72, 2) -> (-72, 5)
  line L15 (-72, 5) -> (-71, 5)
  line L16 (-71, 5) -> (-71, 2)
  line L17 (-71, 2) -> (-57, 2)
  line L18 (-57, 2) -> (-57, 5)
  line L19 (-57, 5) -> (-56, 5)
  line L20 (-56, 5) -> (-56, 2)
  line L21 (-56, 2) -> (-42, 2)
  line L22 (-42, 2) -> (-42, 5)
  line L23 (-42, 5) -> (-41, 5)
  line L24 (-41, 5) -> (-41, 2)
  line L25 (-41, 2) -> (-27, 2)
  line L26 (-27, 2) -> (-27, 5)
  line L27 (-27, 5) -> (-26, 5)
  line L28 (-26, 5) -> (-26, 2)
  line L29 (-26, 2) -> (-12, 2)
  line L30 (-12, 2) -> (-12, 42.5)
  line L31 (-12, 42.5) -> (-131, 42.5)
  line L32 (-117, 5) -> (-116, 5)
  line L33 (-116, 5) -> (-116, 42.5)
  line L34 (-116, 42.5) -> (-117, 42.5)
  line L35 (-117, 42.5) -> (-117, 5)
  constraint horizontal L32
  constraint vertical L33
  constraint horizontal L34
  constraint vertical L35
  constraint coincident L31 L33.end
  constraint coincident L2.end L3.start
extrude "Extrude29" add sketch "Sketch21" along normal blind 3 contours L3 L31 L32 L33 L34 L35
sketch "Sketch22" plane through (0, 12, 0) normal (0, 1, 0) x (-1, 0, 0)
  line L0 (-116, 42.5) -> (-116, 2)
  line L1 (-116, 2) -> (-102, 2)
  line L2 (-102, 2) -> (-102, 5)
  line L3 (-102, 5) -> (-101, 5)
  line L4 (-101, 5) -> (-101, 2)
  line L5 (-101, 2) -> (-87, 2)
  line L6 (-87, 2) -> (-87, 5)
  line L7 (-87, 5) -> (-86, 5)
  line L8 (-86, 5) -> (-86, 2)
  line L9 (-86, 2) -> (-72, 2)
  line L10 (-72, 2) -> (-72, 5)
  line L11 (-72, 5) -> (-71, 5)
  line L12 (-71, 5) -> (-71, 2)
  line L13 (-71, 2) -> (-57, 2)
  line L14 (-57, 2) -> (-57, 5)
  line L15 (-57, 5) -> (-56, 5)
  line L16 (-56, 5) -> (-56, 2)
  line L17 (-56, 2) -> (-42, 2)
  line L18 (-42, 2) -> (-42, 5)
  line L19 (-42, 5) -> (-41, 5)
  line L20 (-41, 5) -> (-41, 2)
  line L21 (-41, 2) -> (-27, 2)
  line L22 (-27, 2) -> (-27, 5)
  line L23 (-27, 5) -> (-26, 5)
  line L24 (-26, 5) -> (-26, 2)
  line L25 (-26, 2) -> (-12, 2)
  line L26 (-12, 2) -> (-12, 42.5)
  line L27 (-12, 42.5) -> (-116, 42.5)
  line L28 (-102, 5) -> (-101, 5)
  line L29 (-101, 5) -> (-101, 42.5)
  line L30 (-101, 42.5) -> (-102, 42.5)
  line L31 (-102, 42.5) -> (-102, 5)
  constraint horizontal L28
  constraint vertical L29
  constraint horizontal L30
  constraint vertical L31
  constraint coincident L27 L29.end
  constraint coincident L2.end L3.start
extrude "Extrude30" add sketch "Sketch22" along normal blind 3 contours L3 L27 L28 L29 L30 L31
sketch "Sketch23" plane through (0, 12, 0) normal (0, 1, 0) x (-1, 0, 0)
  line L0 (-101, 42.5) -> (-101, 2)
  line L1 (-101, 2) -> (-87, 2)
  line L2 (-87, 2) -> (-87, 5)
  line L3 (-87, 5) -> (-86, 5)
  line L4 (-86, 5) -> (-86, 2)
  line L5 (-86, 2) -> (-72, 2)
  line L6 (-72, 2) -> (-72, 5)
  line L7 (-72, 5) -> (-71, 5)
  line L8 (-71, 5) -> (-71, 2)
  line L9 (-71, 2) -> (-57, 2)
  line L10 (-57, 2) -> (-57, 5)
  line L11 (-57, 5) -> (-56, 5)
  line L12 (-56, 5) -> (-56, 2)
  line L13 (-56, 2) -> (-42, 2)
  line L14 (-42, 2) -> (-42, 5)
  line L15 (-42, 5) -> (-41, 5)
  line L16 (-41, 5) -> (-41, 2)
  line L17 (-41, 2) -> (-27, 2)
  line L18 (-27, 2) -> (-27, 5)
  line L19 (-27, 5) -> (-26, 5)
  line L20 (-26, 5) -> (-26, 2)
  line L21 (-26, 2) -> (-12, 2)
  line L22 (-12, 2) -> (-12, 42.5)
  line L23 (-12, 42.5) -> (-101, 42.5)
  line L24 (-87, 5) -> (-86, 5)
  line L25 (-86, 5) -> (-86, 42.5)
  line L26 (-86, 42.5) -> (-87, 42.5)
  line L27 (-87, 42.5) -> (-87, 5)
  constraint horizontal L24
  constraint vertical L25
  constraint horizontal L26
  constraint vertical L27
  constraint coincident L23 L25.end
  constraint coincident L2.end L3.start
extrude "Extrude31" add sketch "Sketch23" along normal blind 3 contours L3 L23 L24 L25 L26 L27
sketch "Sketch24" plane through (0, 12, 0) normal (0, 1, 0) x (-1, 0, 0)
  line L0 (-86, 42.5) -> (-86, 2)
  line L1 (-86, 2) -> (-72, 2)
  line L2 (-72, 2) -> (-72, 5)
  line L3 (-72, 5) -> (-71, 5)
  line L4 (-71, 5) -> (-71, 2)
  line L5 (-71, 2) -> (-57, 2)
  line L6 (-57, 2) -> (-57, 5)
  line L7 (-57, 5) -> (-56, 5)
  line L8 (-56, 5) -> (-56, 2)
  line L9 (-56, 2) -> (-42, 2)
  line L10 (-42, 2) -> (-42, 5)
  line L11 (-42, 5) -> (-41, 5)
  line L12 (-41, 5) -> (-41, 2)
  line L13 (-41, 2) -> (-27, 2)
  line L14 (-27, 2) -> (-27, 5)
  line L15 (-27, 5) -> (-26, 5)
  line L16 (-26, 5) -> (-26, 2)
  line L17 (-26, 2) -> (-12, 2)
  line L18 (-12, 2) -> (-12, 42.5)
  line L19 (-12, 42.5) -> (-86, 42.5)
  line L20 (-72, 5) -> (-71, 5)
  line L21 (-71, 5) -> (-71, 42.5)
  line L22 (-71, 42.5) -> (-72, 42.5)
  line L23 (-72, 42.5) -> (-72, 5)
  constraint horizontal L20
  constraint vertical L21
  constraint horizontal L22
  constraint vertical L23
  constraint coincident L19 L21.end
  constraint coincident L2.end L3.start
extrude "Extrude32" add sketch "Sketch24" along normal blind 3 contours L3 L19 L20 L21 L22 L23
sketch "Sketch25" plane through (0, 12, 0) normal (0, 1, 0) x (-1, 0, 0)
  line L0 (-71, 42.5) -> (-71, 2)
  line L1 (-71, 2) -> (-57, 2)
  line L2 (-57, 2) -> (-57, 5)
  line L3 (-57, 5) -> (-56, 5)
  line L4 (-56, 5) -> (-56, 2)
  line L5 (-56, 2) -> (-42, 2)
  line L6 (-42, 2) -> (-42, 5)
  line L7 (-42, 5) -> (-41, 5)
  line L8 (-41, 5) -> (-41, 2)
  line L9 (-41, 2) -> (-27, 2)
  line L10 (-27, 2) -> (-27, 5)
  line L11 (-27, 5) -> (-26, 5)
  line L12 (-26, 5) -> (-26, 2)
  line L13 (-26, 2) -> (-12, 2)
  line L14 (-12, 2) -> (-12, 42.5)
  line L15 (-12, 42.5) -> (-71, 42.5)
  line L16 (-57, 5) -> (-56, 5)
  line L17 (-56, 5) -> (-56, 42.5)
  line L18 (-56, 42.5) -> (-57, 42.5)
  line L19 (-57, 42.5) -> (-57, 5)
  constraint horizontal L16
  constraint vertical L17
  constraint horizontal L18
  constraint vertical L19
  constraint coincident L15 L17.end
  constraint coincident L2.end L3.start
extrude "Extrude33" add sketch "Sketch25" along normal blind 3 contours L3 L15 L16 L17 L18 L19
sketch "Sketch26" plane through (0, 12, 0) normal (0, 1, 0) x (-1, 0, 0)
  line L0 (-56, 42.5) -> (-56, 2)
  line L1 (-56, 2) -> (-42, 2)
  line L2 (-42, 2) -> (-42, 5)
  line L3 (-42, 5) -> (-41, 5)
  line L4 (-41, 5) -> (-41, 2)
  line L5 (-41, 2) -> (-27, 2)
  line L6 (-27, 2) -> (-27, 5)
  line L7 (-27, 5) -> (-26, 5)
  line L8 (-26, 5) -> (-26, 2)
  line L9 (-26, 2) -> (-12, 2)
  line L10 (-12, 2) -> (-12, 42.5)
  line L11 (-12, 42.5) -> (-56, 42.5)
  line L12 (-42, 5) -> (-41, 5)
  line L13 (-41, 5) -> (-41, 42.5)
  line L14 (-41, 42.5) -> (-42, 42.5)
  line L15 (-42, 42.5) -> (-42, 5)
  dimension "d139" = 1
  constraint horizontal L12
  constraint vertical L13
  constraint horizontal L14
  constraint vertical L15
  constraint coincident L11 L13.end
  constraint coincident L2.end L3.start
  measures "d139" distance of L2.end L3.end
extrude "Extrude34" add sketch "Sketch26" along normal blind 3 contours L3 L11 L12 L13 L14 L15
sketch "Sketch27" plane through (0, 12, 0) normal (0, 1, 0) x (-1, 0, 0)
  line L0 (-41, 42.5) -> (-41, 2)
  line L1 (-41, 2) -> (-27, 2)
  line L2 (-27, 2) -> (-27, 5)
  line L3 (-27, 5) -> (-26, 5)
  line L4 (-26, 5) -> (-26, 2)
  line L5 (-26, 2) -> (-12, 2)
  line L6 (-12, 2) -> (-12, 42.5)
  line L7 (-12, 42.5) -> (-41, 42.5)
  line L8 (-27, 5) -> (-26, 5)
  line L9 (-26, 5) -> (-26, 42.5)
  line L10 (-26, 42.5) -> (-27, 42.5)
  line L11 (-27, 42.5) -> (-27, 5)
  constraint horizontal L8
  constraint vertical L9
  constraint horizontal L10
  constraint vertical L11
  constraint coincident L7 L9.end
  constraint coincident L2.end L3.start
extrude "Extrude35" add sketch "Sketch27" along normal blind 3 contours L3 L7 L8 L9 L10 L11
